snappin (Autodesk Fusion 360 design; units mm, degrees)
Autodesk Fusion 360 part; units mm, degrees
sketch "Sketch1" plane through (0, 0, 0) normal (0, 0, 1) x (1, 0, 0)
  circle A0 centre (0, 0) radius 3.6
  circle A1 centre (0, 0) radius 6
  dimension "d1" = 7.2
  dimension "d2" = 12
  constraint coincident A0.centre A1.centre
  constraint concentric A0 A1
  measures "d1" diameter of A0
  measures "d2" diameter of A1
extrude "Extrude1" add sketch "Sketch1" along normal blind 3.5 contours A0 | A1
extrude "Extrude2" add sketch "Sketch1" along normal blind 38.5 contours A0
sketch "Sketch2" plane through (0, 0, 38.5) normal (0, 0, 1) x (1, 0, 0)
  circle A0 centre (0, 0) radius 3.6
  circle A1 centre (0, 0) radius 3.825
  dimension "d7" = 7.65
  constraint concentric A0 A1
  measures "d7" diameter of A1
extrude "Extrude3" add sketch "Sketch2" along normal blind 3.5 contours A0 | A1
chamfer "Chamfer1" distance 0.225 angle 45 1 edges at (-3.5662, -1.3832, 38.5)
chamfer "Chamfer2" distance 0.35 angle 45 1 edges at (-3.5662, -1.3832, 42)
sketch "Sketch3" plane through (0, 0, 42) normal (0, 0, 1) x (1, 0, 0)
  circle A0 centre (0, 0) radius 3.475
  line L0 (0.2, 3.825) -> (-0.2, 3.825)
  line L1 (-0.2, 3.825) -> (-0.2, -3.825)
  line L2 (-0.2, -3.825) -> (0.2, -3.825)
  line L3 (0.2, -3.825) -> (0.2, 3.825)
  line L4 (0.2, 3.825) -> (-0.2, -3.825) construction
  line L5 (-0.2, 3.825) -> (0.2, -3.825) construction
  line L6 (3.825, -0.2) -> (-3.825, -0.2)
  line L7 (-3.825, -0.2) -> (-3.825, 0.2)
  line L8 (-3.825, 0.2) -> (3.825, 0.2)
  line L9 (3.825, 0.2) -> (3.825, -0.2)
  line L10 (3.825, -0.2) -> (-3.825, 0.2) construction
  line L11 (-3.825, -0.2) -> (3.825, 0.2) construction
  dimension "d12" = 0.4
  dimension "d13" = 7.65
  dimension "d14" = 7.65
  dimension "d15" = 0.4
  constraint horizontal L0
  constraint perpendicular L0 L1
  constraint parallel L0 L2
  constraint parallel L1 L3
  constraint coincident L4 A0.centre
  constraint coincident L5 A0.centre
  constraint coincident A0.centre origin
  constraint horizontal L6
  constraint perpendicular L6 L7
  constraint parallel L6 L8
  constraint parallel L7 L9
  constraint coincident L10 A0.centre
  constraint coincident L11 A0.centre
  measures "d12" distance of L1.end L2.end
  measures "d13" distance of L0.end L1.end
  measures "d14" distance of L7.end L8.end
  measures "d15" distance of L6.end L7.end
extrude "Extrude4" cut sketch "Sketch3" against normal blind 13.5 contours A0 L3 L6 L8 | A0 L6 L8 L9 | A0 L1 L3 L8 | A0 L0 L1 L3 | L1 L3 L6 L8 | A0 L1 L2 L3 | A0 L1 L3 L6 | A0 L1 L6 L8 | A0 L6 L7 L8
equation "d5 = 35 mm + 3.5 mm"
equation "d16 = -10 mm - 3.5 mm"
